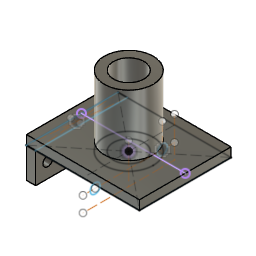
lab1-izvrsni_clan v3 (Autodesk Fusion 360 design; units mm, degrees)
Autodesk Fusion 360 part; units mm, degrees
sketch "Sketch1" plane through (0, 0, 0) normal (0, 0, 1) x (1, 0, 0)
  line L0 (18.5, 15) -> (-18.5, 15)
  line L1 (-18.5, 15) -> (-18.5, -15)
  line L2 (-18.5, -15) -> (18.5, -15)
  line L3 (18.5, -15) -> (18.5, 15)
  line L4 (18.5, 15) -> (-18.5, -15) construction
  line L5 (-18.5, 15) -> (18.5, -15) construction
  circle A0 centre (0, 0) radius 8
  circle A1 centre (0, 0) radius 5
  line L6 (-18.5, 15) -> (-15.5, 15)
  line L7 (-15.5, 15) -> (-15.5, -15)
  line L8 (-15.5, -15) -> (-18.5, -15)
  line L9 (-18.5, -15) -> (-18.5, 15)
  line L10 (-18.5, 15) -> (-15.5, -15) construction
  line L11 (-15.5, 15) -> (-18.5, -15) construction
  line L12 (0, 15) -> (0, -15) construction
  point P0 (-17, 0)
  dimension "d1" = 37
  dimension "d2" = 30
  dimension "d3" = 16
  dimension "d4" = 10
  dimension "d5" = 30
  dimension "d6" = 3
  constraint horizontal L0
  constraint perpendicular L0 L1
  constraint parallel L0 L2
  constraint parallel L1 L3
  constraint coincident L4 A0.centre
  constraint coincident L5 A0.centre
  constraint coincident A0.centre A1.centre
  constraint horizontal L6
  constraint perpendicular L6 L7
  constraint parallel L6 L8
  constraint parallel L7 L9
  constraint coincident L10 P0
  constraint coincident L11 P0
  constraint coincident L0 L1.start
  constraint midpoint L0 L12.start
  constraint midpoint L2 L12.end
  measures "d1" distance of L0.start L0.end
  measures "d2" distance of L0.start L2.end
  measures "d3" diameter of A0
  measures "d4" diameter of A1
  measures "d5" distance of L6.end L7.end
  measures "d6" distance of L7 L9
extrude "Extrude1" add sketch "Sketch1" against normal blind 10 contours L0 L1 L2 L6 L7 L8 L9 makes body 1
extrude "Extrude2" add sketch "Sketch1" along normal blind 3 separate body contours L0 L2 L3 L7 makes body 2
move_body "Move1" bodies 1 to x (1, 0, 0) y (0, 1, 0) z (0, 0, 1) at (3, 0, 0)
extrude "Extrude3" add sketch "Sketch1" along normal blind 23 contours A0 bodies 2
sketch "Sketch2" plane through (0, 0, 0) normal (1, 0, 0) x (0, 1, 0)
  line L0 (15, -5) -> (-15, -5) construction
  line L1 (15, -10) -> (-15, -10) construction
  line L2 (11, 3) -> (11, -10) construction
  line L3 (15, 3) -> (15, -10) construction
  line L4 (0, 3) -> (0, -10) construction
  circle A0 centre (11, -5) radius 1.6
  circle A1 centre (-11, -5) radius 1.6
  dimension "d13" = 5
  dimension "d14" = 13
  dimension "d15" = 4
  dimension "d16" = 3.2
  constraint horizontal L0
  constraint horizontal L1
  constraint coincident L1 L2.end
  constraint perpendicular L1 L2
  constraint perpendicular L1 L3
  constraint midpoint L1 L4.end
  constraint perpendicular L1 L4
  constraint coincident L2 A0.centre
  constraint coincident L0 A0.centre
  constraint symmetric L4 A0 A1
  measures "d13" distance of L0 L1
  measures "d14" distance of L2.start L2.end
  measures "d15" distance of L2 L3
  measures "d16" diameter of A0
extrude "Extrude4" cut sketch "Sketch2" against normal blind 20 contours A1 bodies 1
extrude "Extrude5" cut sketch "Sketch2" against normal blind 35 contours A0 bodies 1
sketch "Sketch3" plane through (0, 0, 0) normal (0, 1, 0) x (1, 0, 0)
  line L0 (-15.5, -3) -> (18.5, -3)
  dimension "d21" = 34
  measures "d21" distance of L0.start L0.end
move_body "Move2" bodies 1 to x (1, 0, 0) y (0, 1, 0) z (0, 0, 1) at (-3, 0, 0)
extrude "Extrude6" add 1 faces at (-15.5, 5, 1) along direction (-1, 0, 0) blind 3 on bodies 2 bodies 1 2
sketch "Sketch4" plane through (0, 0, 0) normal (0, 1, 0) x (1, 0, 0)
sketch "Sketch5" plane through (0, 0, 0) normal (0, 0, 1) x (1, 0, 0)
  line L0 (-16, 0) -> (-19, 0) construction
  constraint horizontal L0
